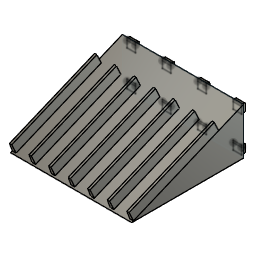
Bobbin_case_holder (Autodesk Fusion 360 design; units mm, degrees)
Autodesk Fusion 360 part; units mm, degrees
sketch "Sketch1" plane through (0, 0, 0) normal (0, 0, 1) x (1, 0, 0)
  line L0 (65, 70) -> (-65, 70)
  line L1 (-65, 70) -> (-65, -70)
  line L2 (-65, -70) -> (65, -70)
  line L3 (65, -70) -> (65, 70)
  line L4 (65, 70) -> (-65, -70) construction
  line L5 (-65, 70) -> (65, -70) construction
  line L6 (-65, -70) -> (65, -70)
  line L7 (65, -70) -> (65, -20)
  line L8 (65, -20) -> (-65, -20)
  line L9 (-65, -20) -> (-65, -70)
  dimension "d1" = 130
  dimension "d2" = 140
  dimension "d3" = 130
  dimension "d4" = 50
  constraint horizontal L0
  constraint perpendicular L0 L1
  constraint parallel L0 L2
  constraint parallel L1 L3
  constraint coincident L4 origin
  constraint coincident L5 origin
  constraint horizontal L6
  constraint vertical L7
  constraint horizontal L8
  constraint vertical L9
  measures "d1" distance of L1.end L2.end
  measures "d2" distance of L0.end L1.end
  measures "d3" distance of L1.end L2.end
  measures "d4" distance of L1.end L8.end
extrude "Extrude1" add sketch "Sketch1" along normal blind 120 contours L1 L2 L3 L6 L7 L8 L9
sketch "Sketch2" plane through (65, 0, 0) normal (1, 0, 0) x (0, 0, -1)
  line L0 (0, -70) -> (0, -20)
  line L1 (0, -20) -> (-120, -20)
  line L2 (-120, -20) -> (-120, -70)
  line L3 (-120, -70) -> (0, -70)
  line L4 (0, -20) -> (-120, -70)
  constraint coincident L0.end L1.start
  constraint coincident L2.end L3.start
extrude "Extrude2" cut sketch "Sketch2" against normal blind 130 contours L1 L2 L4
sketch "Sketch3" plane through (0, -17.0414, -7.1006) normal (0, 0.923077, 0.384615) x (1, 0, 0)
  line L0 (65, -137.6923) -> (65, -7.6923)
  line L1 (65, -7.6923) -> (-65, -7.6923)
  line L2 (-65, -7.6923) -> (-65, -137.6923)
  line L3 (-65, -137.6923) -> (65, -137.6923)
  line L4 (-65, -137.6923) -> (65, -137.6923)
  line L5 (65, -137.6923) -> (65, -135.6923)
  line L6 (65, -135.6923) -> (-65, -135.6923)
  line L7 (-65, -135.6923) -> (-65, -137.6923)
  line L8 (-2, -135.6923) -> (2, -135.6923)
  line L9 (2, -135.6923) -> (2, -36.6923)
  line L10 (2, -36.6923) -> (-2, -36.6923)
  line L11 (-2, -36.6923) -> (-2, -135.6923)
  line L12 (-61, -135.6923) -> (-61, -36.6923)
  line L13 (-65, -36.6923) -> (-65, -135.6923)
  line L14 (-61, -36.6923) -> (-65, -36.6923)
  line L15 (-65, -135.6923) -> (-61, -135.6923)
  line L16 (-40, -135.6923) -> (-40, -36.6923)
  line L17 (-44, -36.6923) -> (-44, -135.6923)
  line L18 (-40, -36.6923) -> (-44, -36.6923)
  line L19 (-44, -135.6923) -> (-40, -135.6923)
  line L20 (-19, -135.6923) -> (-19, -36.6923)
  line L21 (-23, -36.6923) -> (-23, -135.6923)
  line L22 (-19, -36.6923) -> (-23, -36.6923)
  line L23 (-23, -135.6923) -> (-19, -135.6923)
  line L24 (23, -135.6923) -> (23, -36.6923)
  line L25 (19, -36.6923) -> (19, -135.6923)
  line L26 (23, -36.6923) -> (19, -36.6923)
  line L27 (19, -135.6923) -> (23, -135.6923)
  line L28 (44, -135.6923) -> (44, -36.6923)
  line L29 (40, -36.6923) -> (40, -135.6923)
  line L30 (44, -36.6923) -> (40, -36.6923)
  line L31 (40, -135.6923) -> (44, -135.6923)
  line L32 (65, -135.6923) -> (65, -36.6923)
  line L33 (61, -36.6923) -> (61, -135.6923)
  line L34 (65, -36.6923) -> (61, -36.6923)
  line L35 (61, -135.6923) -> (65, -135.6923)
  dimension "d9" = 2
  dimension "d10" = 4
  dimension "d11" = 63
  dimension "d12" = 99
  dimension "d15" = 21
  dimension "d16" = 0
  constraint horizontal L4
  constraint vertical L5
  constraint horizontal L6
  constraint vertical L7
  constraint coincident L2.end L3.start
  constraint horizontal L8
  constraint vertical L9
  constraint horizontal L10
  constraint vertical L11
  constraint collinear L6 L8
  measures "d9" distance of L2.end L6.end
  measures "d10" distance of L9 L11
  measures "d11" distance of L2 L11
  measures "d12" distance of L8 L10
extrude "Extrude3" add sketch "Sketch3" along normal blind 10 contours L0 L6 L32 L33 L34 L35 | L2 L6 L12 L13 L14 L15 | L6 L28 L29 L30 L31 | L6 L16 L17 L18 L19 | L6 L24 L25 L26 L27 | L6 L20 L21 L22 L23 | L6 L8 L9 L10 L11
chamfer "Chamfer1" distance 0.8 distance2 10 14 edges at (-65, -40.9615, 76.3077) (-61, -40.9615, 76.3077) (-44, -40.9615, 76.3077) (-40, -40.9615, 76.3077) (-23, -40.9615, 76.3077) (-19, -40.9615, 76.3077) (-2, -40.9615, 76.3077) (2, -40.9615, 76.3077) (19, -40.9615, 76.3077) (23, -40.9615, 76.3077) (44, -40.9615, 76.3077) (40, -40.9615, 76.3077) (61, -40.9615, 76.3077) (65, -40.9615, 76.3077) measured on face at (-62.3333, -34.6154, 61.0769) measured on face at (-62.3333, -34.6154, 61.0769) measured on face at (-42.6667, -47.3077, 91.5385) measured on face at (-42.6667, -47.3077, 91.5385) measured on face at (-20.3333, -34.6154, 61.0769) measured on face at (-20.3333, -34.6154, 61.0769) measured on face at (-0.6667, -34.6154, 61.0769) measured on face at (-0.6667, -34.6154, 61.0769) measured on face at (21.6667, -47.3077, 91.5385) measured on face at (21.6667, -47.3077, 91.5385) measured on face at (41.3333, -34.6154, 61.0769) measured on face at (41.3333, -34.6154, 61.0769) measured on face at (62.3333, -47.3077, 91.5385) measured on face at (62.3333, -47.3077, 91.5385)
sketch "Sketch5" plane through (0, 0, 0) normal (0, 0, -1) x (-1, 0, 0)
  line L0 (65, -70) -> (65, -20)
  line L1 (65, -20) -> (-65, -20)
  line L2 (-65, -20) -> (-65, -70)
  line L3 (-65, -70) -> (65, -70)
  line L4 (-63, -21) -> (-54, -21)
  line L5 (-54, -21) -> (-54, -30)
  line L6 (-54, -30) -> (-63, -30)
  line L7 (-63, -30) -> (-63, -21)
  line L8 (-16, -30) -> (-25, -30)
  line L9 (-16, -21) -> (-16, -30)
  line L10 (-25, -21) -> (-16, -21)
  line L11 (-25, -30) -> (-25, -21)
  line L12 (22, -30) -> (13, -30)
  line L13 (22, -21) -> (22, -30)
  line L14 (13, -21) -> (22, -21)
  line L15 (13, -30) -> (13, -21)
  line L16 (60, -30) -> (51, -30)
  line L17 (60, -21) -> (60, -30)
  line L18 (51, -21) -> (60, -21)
  line L19 (51, -30) -> (51, -21)
  line L20 (-54, -68) -> (-63, -68)
  line L21 (-54, -59) -> (-54, -68)
  line L22 (-63, -59) -> (-54, -59)
  line L23 (-63, -68) -> (-63, -59)
  line L24 (-16, -68) -> (-25, -68)
  line L25 (-16, -59) -> (-16, -68)
  line L26 (-25, -59) -> (-16, -59)
  line L27 (-25, -68) -> (-25, -59)
  line L28 (22, -68) -> (13, -68)
  line L29 (22, -59) -> (22, -68)
  line L30 (13, -59) -> (22, -59)
  line L31 (13, -68) -> (13, -59)
  line L32 (60, -68) -> (51, -68)
  line L33 (60, -59) -> (60, -68)
  line L34 (51, -59) -> (60, -59)
  line L35 (51, -68) -> (51, -59)
  line L36 (-63, -23) -> (-54, -23)
  line L37 (-25, -23) -> (-16, -23)
  line L38 (13, -23) -> (22, -23)
  line L39 (51, -23) -> (60, -23)
  line L40 (-63, -61) -> (-54, -61)
  line L41 (-25, -61) -> (-16, -61)
  line L42 (13, -61) -> (22, -61)
  line L43 (51, -61) -> (60, -61)
  dimension "d32" = 9
  dimension "d33" = 9
  dimension "d36" = 38
  dimension "d37" = -38
  dimension "d38" = 5
  dimension "d39" = 2
  dimension "d40" = 2
  constraint horizontal L4
  constraint vertical L5
  constraint horizontal L6
  constraint vertical L7
  constraint coincident L7 L36.start
  constraint coincident L5 L36.end
  constraint perpendicular L5 L36
  measures "d32" distance of L4.start L4.end
  measures "d33" distance of L4.start L6.end
  measures "d38" distance of L0 L17
  measures "d39" distance of L3 L20
  measures "d40" distance of L4 L36
extrude "Extrude5" add sketch "Sketch5" along normal blind 4 contours L4 L5 L7 L36 | L9 L10 L11 L37 | L13 L14 L15 L38 | L17 L18 L19 L39 | L21 L22 L23 L40 | L25 L26 L27 L41 | L29 L30 L31 L42 | L33 L34 L35 L43
sketch "Sketch6" plane through (0, -23, 0) normal (0, -1, 0) x (1, 0, 0)
  line L0 (63, 0) -> (54, 0)
  line L1 (54, 0) -> (54, -4)
  line L2 (54, -4) -> (63, -4)
  line L3 (63, -4) -> (63, 0)
  line L4 (63, -4) -> (54, -4)
  line L5 (54, -4) -> (54, -2)
  line L6 (54, -2) -> (63, -2)
  line L7 (63, -2) -> (63, -4)
  line L8 (16, -2) -> (25, -2)
  line L9 (16, -4) -> (16, -2)
  line L10 (25, -4) -> (16, -4)
  line L11 (25, -2) -> (25, -4)
  line L12 (-22, -2) -> (-13, -2)
  line L13 (-22, -4) -> (-22, -2)
  line L14 (-13, -4) -> (-22, -4)
  line L15 (-13, -2) -> (-13, -4)
  line L16 (-60, -2) -> (-51, -2)
  line L17 (-60, -4) -> (-60, -2)
  line L18 (-51, -4) -> (-60, -4)
  line L19 (-51, -2) -> (-51, -4)
  dimension "d43" = 2
  dimension "d46" = -38
  dimension "d47" = 0
  dimension "d58" = 9
  constraint horizontal L4
  constraint vertical L5
  constraint horizontal L6
  constraint vertical L7
  constraint coincident L2.end L3.start
  measures "d43" distance of L4 L6
  measures "d58" distance of L5.end L6.end
sketch "Sketch7" plane through (0, -61, 0) normal (0, -1, 0) x (1, 0, 0)
  line L0 (63, 0) -> (54, 0)
  line L1 (54, 0) -> (54, -4)
  line L2 (54, -4) -> (63, -4)
  line L3 (63, -4) -> (63, 0)
  line L4 (63, -4) -> (54, -4)
  line L5 (54, -4) -> (54, -2)
  line L6 (54, -2) -> (63, -2)
  line L7 (63, -2) -> (63, -4)
  line L8 (16, -2) -> (25, -2)
  line L9 (16, -4) -> (16, -2)
  line L10 (25, -4) -> (16, -4)
  line L11 (25, -2) -> (25, -4)
  line L12 (-22, -2) -> (-13, -2)
  line L13 (-22, -4) -> (-22, -2)
  line L14 (-13, -4) -> (-22, -4)
  line L15 (-13, -2) -> (-13, -4)
  line L16 (-60, -2) -> (-51, -2)
  line L17 (-60, -4) -> (-60, -2)
  line L18 (-51, -4) -> (-60, -4)
  line L19 (-51, -2) -> (-51, -4)
  dimension "d50" = -38
  dimension "d51" = 0
  constraint horizontal L4
  constraint vertical L5
  constraint horizontal L6
  constraint vertical L7
  constraint midpoint L1 L5.end
  constraint coincident L2.end L3.start
extrude "Extrude6" add sketch "Sketch7" along normal blind 7 contours L1 L2 L3 L4 L5 L6 L7 | L8 L9 L10 L11 | L12 L13 L14 L15 | L16 L17 L18 L19
extrude "Extrude7" add sketch "Sketch6" along normal blind 7 contours L1 L2 L3 L4 L5 L6 L7 | L8 L9 L10 L11 | L12 L13 L14 L15 | L16 L17 L18 L19
fillet "Fillet1" radius 1 24 edges at (-55.5, -21, -4) (-17.5, -21, -4) (20.5, -21, -4) (58.5, -21, -4) (58.5, -59, -4) (20.5, -59, -4) (-17.5, -59, -4) (-55.5, -59, -4) (-55.5, -68, -2) (-55.5, -68, -4) (-17.5, -68, -2) (-17.5, -68, -4) (20.5, -68, -2) (20.5, -68, -4) (58.5, -68, -2) (58.5, -68, -4) (58.5, -30, -2) (58.5, -30, -4) (20.5, -30, -2) (20.5, -30, -4) (-17.5, -30, -2) (-17.5, -30, -4) (-55.5, -30, -2) (-55.5, -30, -4)
equation "d11 = ( 130 / 2 ) * 1 mm - 2 mm"
